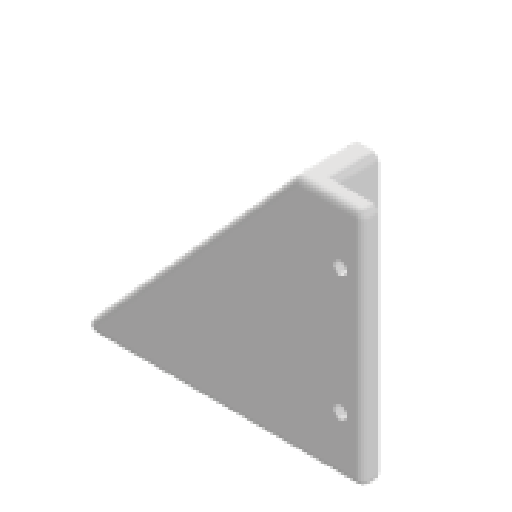
# Autodesk Inventor part: piece of shit number 7
Saved by Autodesk Inventor 2024.1 (Build 281209000, 209)
## iProperties
Created: 2023-08-31
Part Number: piece of shit number 7
Material: Generic
Document SubType Name: Modeling
Designer: mxs6493
Density: 1 g/cm^3
Appearance: Blue - Wall Paint - Glossy
Author: mxs6493
Autodesk Inventor part; units mm, degrees
ref_plane "YZ Plane" through (0, 0, 0) normal (1, 0, 0) x (0, 1, 0)
ref_plane "XZ Plane" through (0, 0, 0) normal (0, 1, 0) x (-1, 0, 0)
ref_plane "XY Plane" through (0, 0, 0) normal (0, 0, 1) x (1, 0, 0)
sketch "Sketch1" plane through (0, 0, 0) normal (0, 0, 1) x (1, 0, 0)
  line L0 (-125, 0) -> (0, 0)
  line L1 (0, 0) -> (0, 105)
  line L2 (0, 105) -> (-30, 105)
  line L3 (-30, 105) -> (-125, 0)
  dimension "d0" = 105
  dimension "d1" = 125
  dimension "d3" = 30
  constraints: 8 end point, 2 horizontal, 1 coincident, 1 vertical
  measures "d0" distance of L0.end L1.end
  measures "d1" distance of L0.start L0.end
  measures "d3" distance of L1.end L2.end
extrude "Extrusion1" add sketch "Sketch1" along normal blind 7
sketch "Sketch2" plane through (0, 0, 0) normal (0, 0, -1) x (-1, 0, 0)
  line L0 (0, 105) -> (30, 105) projected
  line L1 (20, 105) -> (20, 0)
  line L2 (125, 0) -> (0, 0) projected
  line L3 (0, 0) -> (0, 105) projected
  line L4 (125, 0) -> (0, 0) projected
  line L5 (30, 105) -> (125, 0) projected
  line L6 (0, 105) -> (30, 105) projected
  line L7 (20, 0) -> (125, 0)
  line L8 (20, 105) -> (30, 105)
  line L9 (30, 105) -> (125, 0)
  line L10 (25, 5) -> (25, 100)
  line L11 (25, 100) -> (27.781, 100)
  line L12 (27.781, 100) -> (113.7334, 5)
  line L13 (113.7334, 5) -> (25, 5)
  dimension "d6" = 20
  dimension "d7" = 5
  constraints: 16 end point, 3 collinear, 2 point on line, 1 vertical, 3 other
  measures "d6" distance between parallel lines of L3 L1
  measures "d7" distance between parallel lines of L1 L10
extrude "Extrusion2" add sketch "Sketch2" along normal blind 20 contours L0 L5 L2 L1
fillet "Fillet1" radius 3 14 edges at (-20, 0, -10) (-20, 105, -10) (-30, 105, -6.5) (-125, 0, -6.5) (0, 0, 3.5) (0, 105, 3.5) (-27.781, 100, -10) (-25, 100, -10) (-25, 5, -10) (-113.7334, 5, -10) (-77.5, 52.5, 7) (-62.5, 0, 7) (0, 52.5, 7) (-15, 105, 7)
sketch "Sketch3" plane through (0, 0, 0) normal (0, 0, -1) x (-1, 0, 0)
  line L0 (23, 0) -> (0, 0) projected
  line L1 (0, 0) -> (0, 102) projected
  line L2 (3, 105) -> (23, 105) projected
  point P0 (10, 25)
  point P1 (10, 80)
  point P2 (3, 0)
  point P3 (0, 3)
  point P4 (20, 0)
  point P5 (0, 105)
  point P6 (20, 105)
  dimension "d18" = 25
  dimension "d19" = 10
  dimension "d23" = 55
  constraints: 1 vertical alignment
  measures "d18" distance from line of L0 point (10, 25)
  measures "d19" distance from line of L1 point (10, 25)
  measures "d23" distance of point (10, 80) point (10, 25)
hole "Hole1" at (-10, 25, 0) at (-10, 80, 0) direction (0, 0, 1) diameter 5.8 end through all clearance for "Flat Head Machine Screw" size "M5" standard "Ansi Metric M Profile"
sketch "Sketch5" plane through (-125, 0, -20) normal (-0.7415358, 0.6709133, 0) x (0, 0, 1)
  line L0 (0, 141.598) -> (27, 141.598) projected
  line L1 (0, 6.7599) -> (0, 140.2667) projected
  line L2 (0, 73.5133) -> (23.5837, 73.5133) construction
  line L3 (24, 6.7599) -> (0, 6.7599) projected
  line L4 (24, 140.2667) -> (24, 6.7599) projected
  line L5 (0, 140.2667) -> (24, 140.2667) projected
  point P0 (20, 83.8642)
  point P1 (10, 41.0133)
  point P2 (10, 106.0133)
  dimension "d38" = 65
  dimension "d40" = 10
  constraints: 2 end point, 1 horizontal, 1 midpoint, 1 symmetric about line
  measures "d38" distance of point (10, 41.013) point (10, 106.013)
  measures "d40" distance from line of L1 point (10, 41.013)
hole "Hole3" at (-97.4836, 30.4128, -10) at (-53.8743, 78.6127, -10) direction (0.7415358, -0.6709133, 0) diameter 5.8 depth 5 tip angle 118 clearance for "Flat Head Machine Screw" size "M5" standard "Ansi Metric M Profile"
body "Solid1"
